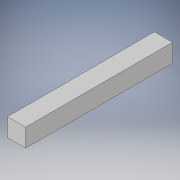
# Autodesk Inventor part: LinearExample
Saved by Autodesk Inventor 2017 (Build 210142000, 142)
## iProperties
Created: 2016-05-08
Part Number: LinearExample
Material: Generic
Document SubType Name: Modeling
Designer: steele
Density: 1 g/cm^3
Appearance: Default
Author: steele
Autodesk Inventor part; units mm, degrees
ref_plane "YZ Plane" through (0, 0, 0) normal (1, 0, 0) x (0, 1, 0)
ref_plane "XZ Plane" through (0, 0, 0) normal (0, 1, 0) x (-1, 0, 0)
ref_plane "XY Plane" through (0, 0, 0) normal (0, 0, 1) x (1, 0, 0)
sketch "Sketch1" plane through (0, 0, 0) normal (0, 0, 1) x (1, 0, 0)
  line L0 (-19.05, -19.05) -> (19.05, -19.05)
  line L1 (19.05, -19.05) -> (19.05, 19.05)
  line L2 (19.05, 19.05) -> (-19.05, 19.05)
  line L3 (-19.05, 19.05) -> (-19.05, -19.05)
  line L4 (-19.05, -19.05) -> (19.05, 19.05) construction
  line L5 (19.05, -19.05) -> (-19.05, 19.05) construction
  line L6 (-15.875, -15.875) -> (15.875, -15.875)
  line L7 (15.875, -15.875) -> (15.875, 15.875)
  line L8 (15.875, 15.875) -> (-15.875, 15.875)
  line L9 (-15.875, 15.875) -> (-15.875, -15.875)
  line L10 (-15.875, -15.875) -> (15.875, 15.875) construction
  line L11 (15.875, -15.875) -> (-15.875, 15.875) construction
  point P0 (0, 0)
  dimension "d0" = 38.1
  dimension "d1" = 3.175
  constraints: 24 end point, 4 midpoint, 4 parallel, 4 perpendicular, 2 horizontal
  measures "d0" distance of L2.end L0.start
  measures "d1" distance between parallel lines of L3 L9
extrude "Extrusion1" add sketch "Sketch1" along normal mid plane 304.8
sketch "Sketch3" plane through (0, 0, 152.4) normal (0, 0, 1) x (1, 0, 0)
  line L0 (-19.05, -19.05) -> (19.05, -19.05)
  line L1 (19.05, -19.05) -> (19.05, 19.05)
  line L2 (19.05, 19.05) -> (-19.05, 19.05)
  line L3 (-19.05, 19.05) -> (-19.05, -19.05)
  line L4 (-19.05, -19.05) -> (19.05, 19.05) construction
  line L5 (19.05, -19.05) -> (-19.05, 19.05) construction
  point P0 (0, 0)
  constraints: 12 end point, 2 midpoint, 2 parallel, 2 perpendicular
extrude "Extrusion2" add sketch "Sketch3" along normal blind 3.175
body "Solid1"
